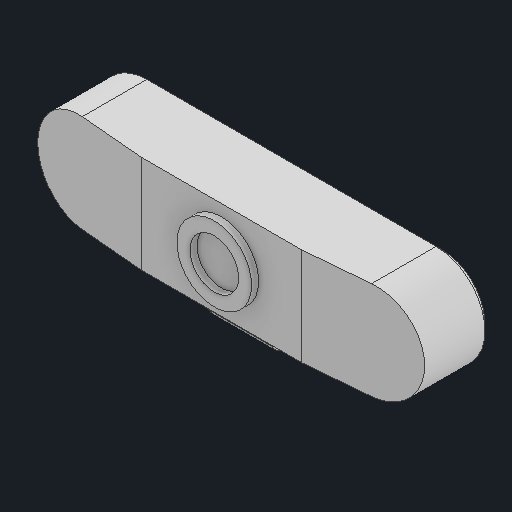
# Autodesk Inventor part: Emeet_Camera
Saved by Autodesk Inventor 2024 (Build 280153000, 153)
## iProperties
Created: 2025-09-16
Part Number: Emeet_Camera
Material: Generic
Document SubType Name: Modeling
Designer: kevin
Density: 1 g/cm^3
Appearance: Default
Author: kevin
Autodesk Inventor part; units mm, degrees
ref_plane "YZ Plane" through (0, 0, 0) normal (1, 0, 0) x (0, 1, 0)
ref_plane "XZ Plane" through (0, 0, 0) normal (0, 1, 0) x (-1, 0, 0)
ref_plane "XY Plane" through (0, 0, 0) normal (0, 0, 1) x (1, 0, 0)
sketch "Sketch1" plane through (0, 0, 0) normal (0, 0, 1) x (1, 0, 0)
  line L0 (-62, -15.65) -> (62, -15.65)
  line L1 (62, -15.65) -> (62, 15.65)
  line L2 (62, 15.65) -> (-62, 15.65)
  line L3 (-62, 15.65) -> (-62, -15.65)
  line L4 (-62, -15.65) -> (62, 15.65) construction
  line L5 (62, -15.65) -> (-62, 15.65) construction
  line L6 (-62, 0) -> (62, 0) construction
  line L7 (-46.35, -15.65) -> (46.35, -15.65)
  line L8 (46.35, 15.65) -> (-46.35, 15.65)
  arc A0 (-46.35, 15.65) -> (-46.35, -15.65) centre (-46.35, 0) ccw
  arc A1 (46.35, -15.65) -> (46.35, 15.65) centre (46.35, 0) ccw
  point P0 (0, 0)
  point P1 (0, 0)
  point P2 (-62, 0)
  point P3 (-46.35, 15.65)
  point P4 (62, 0)
  point P5 (46.35, -15.65)
  dimension "d0" = 124
  dimension "d1" = 31.3
  constraints: 20 end point, 6 point on circle, 5 midpoint, 4 tangent, 3 parallel, 2 centre point, 2 point on line, 1 horizontal, 1 perpendicular
  measures "d0" distance of L2.end L1.end
  measures "d1" distance of L1.end L0.end
extrude "Extrusion1" add sketch "Sketch1" along normal blind 24.5
sketch "Sketch2" plane through (0, 0, 24.5) normal (0, 0, 1) x (1, 0, 0)
  circle A0 centre (0, 0) radius 11.975
  circle A1 centre (0, 0) radius 7.8185
  dimension "d4" = 23.95
  constraints: 2 centre point, 1 coincident
  measures "d4" diameter of A0
extrude "Extrusion2" add sketch "Sketch2" along normal blind 2.25
chamfer "Chamfer1" distance 3.175 angle 85 1 edges at (62, 0, 24.5) measured on face at (62, -5.2167, 8.1667)
chamfer "Chamfer2" distance 3.175 angle 85 1 edges at (-62, 0, 24.5) measured on face at (-62, 5.2167, 8.1667)
extrude "Extrusion3" cut sketch "Sketch1" along normal blind 24.5 contours L3 A0 L0 | L3 L2 A0 | A1 L1 L0 | A1 L2 L1
chamfer "Chamfer3" distance 2 angle 45 2 edges at (62, 0, 0) (-62, 0, 0)
sketch "Sketch4" plane through (0, 0, 0) normal (1, 0, 0) x (0, 1, 0)
  line L0 (15.65, 24.5) -> (-15.65, 24.5) construction
  line L1 (-15.65, 24.5) -> (-15.65, 0) construction
  line L2 (-15.65, 10.6) -> (-24.65, 10.6)
  line L3 (-24.65, 10.6) -> (-24.65, 18.35)
  line L4 (-24.65, 18.35) -> (-15.65, 18.35)
  line L5 (-15.65, 18.35) -> (-15.65, 10.6)
  circle A0 centre (-20.5, 14.475) radius 2.25
  arc A1 (-21.9856, 18.35) -> (-21.9856, 10.6) centre (-20.5, 14.475) ccw
  line L6 (-15.65, 14.475) -> (-24.65, 14.475) construction
  point P0 (0, 0)
  point P1 (-13.65, 0)
  point P2 (-15.65, 2)
  dimension "d19" = 10.6
  dimension "d20" = 9
  dimension "d21" = 7.75
  dimension "d22" = 4.5
  dimension "d23" = 1.9
  constraints: 12 end point, 4 point on line, 2 centre point, 2 midpoint, 2 parallel, 2 point on circle, 1 horizontal, 1 perpendicular, 1 tangent, 1 vertical
  measures "d19" distance from line of L1.end L2
  measures "d20" distance of L2.start L2.end
  measures "d21" distance of L2.end L3.end
  measures "d22" diameter of A0
  measures "d23" radial gap between concentric circles of A0 A1
extrude "Extrusion4" add sketch "Sketch4" along normal mid plane 20.2 contours L2 A1 L4 L5
body "Solid1"
